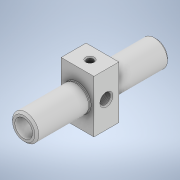
# Autodesk Inventor part: Колонка-1
Saved by Autodesk Inventor 2022 (Build 260153000, 153)
## iProperties
Created: 2021-12-03
Part Number: Колонка-1
Material: Типовые
Document SubType Name: Modeling
Designer: Украинцев
Density: 1 g/cm^3
Appearance: По умолчанию
Author: Украинцев
Autodesk Inventor part; units mm, degrees
note: some values were not read from the file. Chosen so that the rebuilt part matches the saved one: direction of "Отверстие2"; direction of "Отверстие3"; direction of "Отверстие4".
ref_plane "YZ Plane" through (0, 0, 0) normal (1, 0, 0) x (0, 1, 0)
ref_plane "XZ Plane" through (0, 0, 0) normal (0, 1, 0) x (-1, 0, 0)
ref_plane "XY Plane" through (0, 0, 0) normal (0, 0, 1) x (1, 0, 0)
sketch "Эскиз1" plane through (0, 0, 0) normal (0, 1, 0) x (-1, 0, 0)
  line L0 (0, 0) -> (0, 101)
  line L1 (0, 101) -> (20, 101)
  line L2 (20, 101) -> (20, -101)
  line L3 (20, -101) -> (0, -101)
  line L4 (0, -101) -> (0, 0)
  line L5 (-25, 19) -> (25, 19)
  line L6 (25, 19) -> (25, -19)
  line L7 (25, -19) -> (-25, -19)
  line L8 (-25, -19) -> (-25, 19)
  line L9 (-25, 19) -> (25, -19) construction
  line L10 (25, 19) -> (-25, -19) construction
  line L11 (20, 19) -> (20, 22)
  line L12 (0, 19) -> (19.75, 19)
  line L13 (19.75, 19) -> (19.75, 22)
  line L14 (19.75, 22) -> (20, 22)
  line L15 (19.75, 19) -> (20.75, 19)
  line L16 (20.75, 19) -> (20.75, 20)
  circle A0 centre (20.75, 20) radius 1
  line L17 (20, 22) -> (19.75, 20)
  line L18 (20, -19) -> (20, -22)
  line L19 (20, -22) -> (19.754, -22)
  line L20 (19.754, -22) -> (19.754, -19)
  line L21 (19.754, -19) -> (20.754, -19)
  line L22 (20.754, -19) -> (20.754, -20)
  line L23 (20.754, -20) -> (19.754, -20)
  line L24 (19.754, -20) -> (19.754, -19)
  circle A1 centre (20.754, -20) radius 1
  line L25 (19.754, -20) -> (20, -22)
  point P0 (0, -19)
  point P1 (19.7838, -20.2423)
  point P2 (19.7808, 20.2462)
  dimension "d0" = 101
  dimension "d1" = 20
  dimension "d2" = 202
  dimension "d3" = 50
  dimension "d4" = 38
  dimension "d8" = 3
  dimension "d9" = 19.75
  dimension "d10" = 1
  dimension "d11" = 1
  dimension "d12" = 3
  dimension "d13" = 0.246
  dimension "d14" = 1
  dimension "d15" = 1
  constraints: 52 end point, 11 point on line, 9 perpendicular, 5 parallel, 3 horizontal, 3 midpoint, 2 coincident, 2 point on circle, 1 centre point, 1 vertical, 3 other
  measures "d0" distance of L0.start L0.end
  measures "d1" distance of L0.end L1.end
  measures "d2" distance of L1.end L2.end
  measures "d3" distance of L6.end L7.end
  measures "d4" distance of L5.end L6.end
  measures "d8" distance of L11.start L11.end
  measures "d9" distance of L12.start L12.end
  measures "d10" distance of L12.end L15.end
  measures "d11" distance of L15.end L16.end
  measures "d12" distance of L18.start L18.end
  measures "d13" distance of L18.end L19.end
  measures "d14" distance of L22.end L23.end
  measures "d15" distance of L21.end L22.end
extrude "Выдавливание1" add sketch "Эскиз1" along normal mid plane 80 contours L4 L7 L8 L5 L0 | L0 L5 L2 L7 L4 | L5 L6 L7 L2
revolve "Вращение1" add sketch "Эскиз1" angle 360 about axis through (0, 0, 0) along (0, 0, 1) contours L0 L1 L2 L14 L13 L5 | L7 L20 L19 L2 L3 L4 | L13 A0 L2 L5 | L7 L2 A1 L20 | L2 A0 L5 | L13 L14 L17 A0 | L7 A1 L2 | A1 L25 L19 L20
sketch "Эскиз2" plane through (0, 0, -101) normal (0, 0, -1) x (-1, 0, 0)
  point P0 (0, 0)
  point P1 (0, 0)
  constraints: 1 coincident
hole "Отверстие1" at (0, 0, -101) direction (0, 0, 1) diameter 27 end through all
sketch "Эскиз3" plane through (0, -40, 0) normal (0, -1, 0) x (1, 0, 0)
  point P0 (0, 0)
  point P1 (0, 0)
  constraints: 1 coincident
hole "Отверстие2" at (0, -40, 0) direction (0, 1, 0) diameter 24 end up to surface
sketch "Эскиз4" plane through (0, 40, 0) normal (0, 1, 0) x (1, 0, 0)
  point P0 (0, 0)
  point P1 (0, 0)
  constraints: 1 coincident
hole "Отверстие3" at (0, 40, 0) direction (0, -1, 0) diameter 10 end up to surface
sketch "Эскиз5" plane through (25, -40, -19) normal (1, 0, 0) x (0, 0, -1)
  point P0 (-19, 40)
  point P1 (-19, 40)
  constraints: 1 coincident
hole "Отверстие4" at (25, 0, 0) direction (-1, 0, 0) diameter 16 end up to surface
sketch "Эскиз6" plane through (0, -40, 0) normal (0, -1, 0) x (1, 0, 0)
  line L0 (16, -12) -> (-16, -12)
  line L1 (-16, -12) -> (-16, 12)
  line L2 (-16, 12) -> (16, 12)
  line L3 (16, 12) -> (16, -12)
  line L4 (16, -12) -> (-16, 12) construction
  line L5 (-16, -12) -> (16, 12) construction
  point P0 (0, 0)
  dimension "d44" = 32
  dimension "d45" = 24
  constraints: 12 end point, 3 coincident, 2 midpoint, 2 parallel, 1 horizontal, 1 perpendicular
  measures "d44" distance of L1.end L2.end
  measures "d45" distance of L0.end L1.end
hole "Отверстие5" at (16, -40, -12) at (-16, -40, 12) direction (0, 1, 0) diameter 6 depth 14 tip angle 118
hole "Отверстие6" at (16, -40, 12) direction (0, 1, 0) diameter 8 depth 22 tip angle 118
chamfer "Фаска1" distance 2 angle 45 1 edges at (25, 0, 8)
chamfer "Фаска2" distance 1.6 angle 45 1 edges at (16, -40, 16)
thread "Резьба1" size "M6x1" class "6H" standard "ANSI Metric M Profile" length 9
thread "Резьба2" size "M6x1" class "6H" standard "ANSI Metric M Profile" length 9
chamfer "Фаска3" distance 1 angle 45 2 edges at (-16, -40, 15) (16, -40, -9)
thread "Резьба3" size "M10x1.5" class "6H" standard "ANSI Metric M Profile" full length
chamfer "Фаска4" distance 1.6 angle 45 1 edges at (0, 40, -5)
thread "Резьба4" size "M16x2" class "6H" standard "ANSI Metric M Profile" full length
chamfer "Фаска5" distance 3 angle 45 2 edges at (20, 0, 101) (20, 0, -101)
